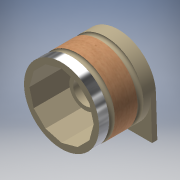
# Autodesk Inventor part: mounting plate
Saved by Autodesk Inventor 2017 (Build 210142000, 142)
## iProperties
Created: 2017-11-23
Part Number: mounting plate
Material: ABS Plastic
Document SubType Name: Modeling
Designer: prakh
Density: 1.06 g/cm^3
Appearance: Beige
Author: prakh
Autodesk Inventor part; units mm, degrees
ref_plane "YZ Plane" through (0, 0, 0) normal (1, 0, 0) x (0, 1, 0)
ref_plane "XZ Plane" through (0, 0, 0) normal (0, 1, 0) x (-1, 0, 0)
ref_plane "XY Plane" through (0, 0, 0) normal (0, 0, 1) x (1, 0, 0)
sketch "Sketch1" plane through (0, 0, 0) normal (0, 0, 1) x (1, 0, 0)
  circle A0 centre (0, 0) radius 47.625
  line L0 (-47.625, 47.625) -> (47.625, 47.625)
  line L1 (47.625, 47.625) -> (47.625, -47.625)
  line L2 (47.625, -47.625) -> (-47.625, -47.625)
  line L3 (-47.625, -47.625) -> (-47.625, 47.625)
  dimension "d0" = 95.25
  dimension "d1" = 95.25
  dimension "d2" = 95.25
  dimension "d3" = 47.625
  dimension "d4" = 47.625
  constraints: 8 end point, 2 parallel, 1 centre point, 1 coincident, 1 horizontal, 1 perpendicular
  measures "d0" diameter of A0
  measures "d1" distance of L1.end L2.end
  measures "d2" distance of L0.end L1.end
  measures "d3" distance from line of point (0, 0) L1
  measures "d4" distance from line of point (0, 0) L0
extrude "Extrusion1" add sketch "Sketch1" along normal blind 6.35
sketch "Sketch2" plane through (0, 0, 6.35) normal (0, 0, 1) x (1, 0, 0)
  circle A0 centre (0, 0) radius 47.625
  circle A1 centre (0, 0) radius 46.0375
  line L0 (0, 39.444) -> (19.722, 34.1595)
  line L1 (19.722, 34.1595) -> (34.1595, 19.722)
  line L2 (34.1595, 19.722) -> (39.444, 0)
  line L3 (39.444, 0) -> (34.1595, -19.722)
  line L4 (34.1595, -19.722) -> (19.722, -34.1595)
  line L5 (19.722, -34.1595) -> (0, -39.444)
  line L6 (0, -39.444) -> (-19.722, -34.1595)
  line L7 (-19.722, -34.1595) -> (-34.1595, -19.722)
  line L8 (-34.1595, -19.722) -> (-39.444, 0)
  line L9 (-39.444, 0) -> (-34.1595, 19.722)
  line L10 (-34.1595, 19.722) -> (-19.722, 34.1595)
  line L11 (-19.722, 34.1595) -> (0, 39.444)
  dimension "d7" = 95.25
  dimension "d8" = 1.5875
  dimension "d25" = 76.2
  constraints: 24 end point, 3 coincident, 2 centre point, 25 other
  measures "d7" diameter of A0
  measures "d8" radial gap between concentric circles of A1 A0
  measures "d25" distance between parallel lines of L5 L11
extrude "Extrusion2" add sketch "Sketch2" along normal blind 63.5 contours A1
sketch "Sketch3" plane through (0, 0, 6.35) normal (0, 0, 1) x (1, 0, 0)
  circle A0 centre (0, 0) radius 14.2875
  dimension "d11" = 28.575
  constraints: 1 centre point, 1 coincident
  measures "d11" diameter of A0
extrude "Extrusion3" cut sketch "Sketch3" against normal blind 38.1
sketch "Sketch4" plane through (0, 0, 6.35) normal (0, 0, 1) x (1, 0, 0)
  circle A0 centre (0, 0) radius 14.2875 projected
  circle A1 centre (0, 0) radius 19.05
  dimension "d14" = 38.1
  constraints: 1 centre point, 1 coincident
  measures "d14" diameter of A1
extrude "Extrusion4" add sketch "Sketch4" along normal blind 34.925
sketch "Sketch6" plane through (0, 0, 6.35) normal (0, 0, 1) x (1, 0, 0)
  circle A0 centre (31.75, 0) radius 6.35
  point P0 (0, 0)
  dimension "d21" = 12.7
  dimension "d22" = 31.75
  constraints: 1 centre point, 1 horizontal alignment
  measures "d21" diameter of A0
  measures "d22" distance of point (0, 0) A0.centre
extrude "Extrusion6" cut sketch "Sketch6" against normal blind 25.4
sketch "Sketch7" plane through (0, 0, 6.35) normal (0, 0, 1) x (1, 0, 0)
  line L0 (47.625, 47.625) -> (-47.625, 47.625) projected
  line L1 (-47.625, 47.625) -> (-47.625, -47.625) projected
  line L2 (-47.625, -47.625) -> (47.625, -47.625) projected
  line L3 (47.625, -47.625) -> (47.625, 47.625) projected
  circle A0 centre (0, 0) radius 46.0375 projected
  line L4 (47.625, -47.625) -> (47.625, 47.625) projected
  circle A1 centre (0, 0) radius 46.0375 projected
  line L5 (-47.625, -47.625) -> (-46.0127, 1.5098)
  line L6 (47.625, -47.625) -> (46.0127, 1.5098)
  point P0 (-46.0127, -1.5098)
  point P1 (46.0127, -1.5098)
  constraints: 4 end point, 4 point on circle, 2 tangent
extrude "Extrusion7" cut sketch "Sketch7" against normal blind 25.4 contours L3 L6 A0 L5 L1 L0
sketch "Sketch8" plane through (0, 0, 0) normal (0, 1, 0) x (-1, 0, 0)
  line L0 (46.0375, 6.35) -> (46.0375, 69.85) projected
  arc A0 (46.0375, 57.5151) -> (46.0375, 50.4349) centre (45.0215, 53.975) ccw
  arc A1 (46.0375, 22.5901) -> (46.0375, 15.5099) centre (45.0215, 19.05) ccw
  line L1 (46.0375, 69.85) -> (-46.0375, 69.85) projected
  line L2 (0, -13.97) -> (0, 83.82) projected
  arc A2 (45.0215, 15.367) -> (46.0375, 22.5901) centre (45.0215, 19.05) ccw
  point P0 (0, 0)
  dimension "d28" = 3.683
  dimension "d31" = 12.7
  dimension "d32" = 15.875
  dimension "d34" = 2.667
  constraints: 6 point on circle, 4 point on line, 3 centre point, 1 coincident, 1 equal radius, 1 vertical alignment
  measures "d28" radius of A1
  measures "d31" vertical distance of L0.start A1.centre
  measures "d32" distance from line of A0.centre L1
  measures "d34" distance edge to line of A2 L0
revolve "Revolution1" cut sketch "Sketch8" angle 360 about axis through (0, 0, -10) along (0, 0, 1) contours A1 L0 | A0 L0
sketch "Sketch9" plane through (0, 0, 6.35) normal (0, 0, 1) x (1, 0, 0)
  circle A0 centre (31.75, 0) radius 6.35 projected
  circle A1 centre (0, 0) radius 19.05 projected
  line L0 (34.1595, 19.722) -> (19.722, 34.1595) projected
  line L1 (19.722, 34.1595) -> (0, 39.444) projected
  line L2 (0, 39.444) -> (-19.722, 34.1595) projected
  line L3 (-19.722, 34.1595) -> (-34.1595, 19.722) projected
  line L4 (-34.1595, 19.722) -> (-39.444, 0) projected
  line L5 (-39.444, 0) -> (-34.1595, -19.722) projected
  line L6 (-34.1595, -19.722) -> (-19.722, -34.1595) projected
  line L7 (-19.722, -34.1595) -> (0, -39.444) projected
  line L8 (0, -39.444) -> (19.722, -34.1595) projected
  line L9 (19.722, -34.1595) -> (34.1595, -19.722) projected
  line L10 (34.1595, -19.722) -> (39.444, 0) projected
  line L11 (39.444, 0) -> (34.1595, 19.722) projected
  circle A2 centre (0, -31.75) radius 4.826
  dimension "d35" = 9.652
  dimension "d36" = 31.75
  dimension "d37" = 31.75
  constraints: 1 centre point, 1 vertical alignment
  measures "d35" diameter of A2
  measures "d36" distance of point (0, 0) A0.centre
  measures "d37" distance of A2.centre point (0, 0)
extrude "Extrusion8" cut sketch "Sketch9" against normal blind 25.4 contours A2
sketch "Sketch10" plane through (0, 0, 6.35) normal (0, 0, 1) x (1, 0, 0)
  circle A0 centre (0, -31.75) radius 4.826 projected
  circle A1 centre (31.75, 0) radius 6.35 projected
  circle A2 centre (0, 0) radius 19.05 projected
  line L0 (34.1595, 19.722) -> (19.722, 34.1595) projected
  line L1 (19.722, 34.1595) -> (0, 39.444) projected
  line L2 (0, 39.444) -> (-19.722, 34.1595) projected
  line L3 (-19.722, 34.1595) -> (-34.1595, 19.722) projected
  line L4 (-34.1595, 19.722) -> (-39.444, 0) projected
  line L5 (-39.444, 0) -> (-34.1595, -19.722) projected
  line L6 (-34.1595, -19.722) -> (-19.722, -34.1595) projected
  line L7 (-19.722, -34.1595) -> (0, -39.444) projected
  line L8 (0, -39.444) -> (19.722, -34.1595) projected
  line L9 (19.722, -34.1595) -> (34.1595, -19.722) projected
  line L10 (34.1595, -19.722) -> (39.444, 0) projected
  line L11 (39.444, 0) -> (34.1595, 19.722) projected
  arc A3 (7.6781, -37.3867) -> (-7.6781, -37.3867) centre (0, -31.75) ccw
  dimension "d40" = 19.05
  constraints: 2 point on circle, 2 point on line, 1 centre point, 1 coincident
  measures "d40" diameter of A3
extrude "Extrusion9" cut sketch "Sketch10" against normal blind 3.175 contours L8 L7 A3
sketch "Sketch11" plane through (0, 0, 0) normal (0, 1, 0) x (-1, 0, 0)
  line L0 (-19.05, 6.35) -> (-19.05, 41.275) projected
  line L1 (-19.05, 38.1) -> (-26.605, 25.4)
  line L2 (-26.605, 25.4) -> (-23.8011, 25.4)
  line L3 (46.0375, 22.5901) -> (-46.0375, 22.5901) projected
  line L4 (-23.8011, 25.4) -> (-17.684, 35.6829)
  point P0 (0, 0)
  dimension "d43" = 25.4
  dimension "d44" = 12.7
  constraints: 6 end point, 2 parallel, 1 point on line
  measures "d43" distance from line of point (0, 0) L2
  measures "d44" vertical distance of L1.start L1.end
equation "\"d3\" = 0.5 * d1"
equation "\"d4\" = 0.5 * d2"
equation "\"d37\" = d36"
body "Solid1"
